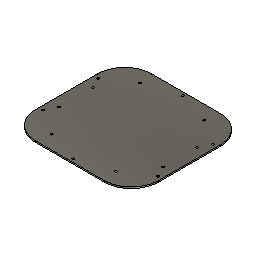
バスケット底 v3 (Autodesk Fusion 360 design; units mm, degrees)
Autodesk Fusion 360 part; units mm, degrees
note: some values were not read from the file. Set by a fixed rule: which sketch regions a step uses.
sketch "スケッチ1" plane through (0, 0, 0) normal (0, 0, 1) x (1, 0, 0)
  circle A0 centre (0, 0) radius 75
  circle A1 centre (0, 0) radius 85
  line L0 (0, 75) -> (0, 85)
  circle A2 centre (0, 80) radius 1.6
  circle A3 centre (-47.0228, 64.7214) radius 1.6
  circle A4 centre (-76.0845, 24.7214) radius 1.6
  circle A5 centre (-76.0845, -24.7214) radius 1.6
  circle A6 centre (-47.0228, -64.7214) radius 1.6
  circle A7 centre (0, -80) radius 1.6
  circle A8 centre (47.0228, -64.7214) radius 1.6
  circle A9 centre (76.0845, -24.7214) radius 1.6
  circle A10 centre (76.0845, 24.7214) radius 1.6
  circle A11 centre (47.0228, 64.7214) radius 1.6
  line L1 (0, 0) -> (-84, 0)
  line L2 (-84, 0) -> (-84, -40.186)
  line L3 (0, 0) -> (0, 85)
  line L4 (84, 0) -> (84, -40.186)
  line L5 (-84, 0) -> (-84, 40.186)
  line L6 (84, 0) -> (84, 40.186)
  circle A12 centre (-84, 40.186) radius 1.6
  circle A13 centre (84, 40.186) radius 1.6
  circle A14 centre (-84, -40.186) radius 1.6
  circle A15 centre (84, -40.186) radius 1.6
  line L7 (0, 85) -> (-90, 85)
  line L8 (-90, 85) -> (-90, 0)
  line L9 (-90, 0) -> (0, 0)
  line L10 (0, 0) -> (0, 85)
  line L11 (90, 85) -> (90, 0)
  line L12 (0, 85) -> (90, 85)
  line L13 (-90, -85) -> (-90, 0)
  line L14 (0, -85) -> (-90, -85)
  line L15 (0, -85) -> (90, -85)
  line L16 (90, -85) -> (90, 0)
  dimension "d1" = 150
  dimension "d4" = 170
  dimension "d7" = 3.2
  dimension "d9" = 360
  dimension "d10" = 84
  dimension "d11" = 40.186
  dimension "d12" = 3.2
  dimension "d13" = 3.2
  dimension "d14" = 3.2
  dimension "d15" = 3.2
  constraint coincident A0.centre A1.centre
  constraint concentric A0 A1
  constraint coincident A0 L0.start
  constraint coincident A1 L0.end
  constraint vertical L0
  constraint midpoint L0 A2.centre
  constraint horizontal L1
  constraint perpendicular L1 L2
  constraint parallel L0 L3
  constraint symmetric L1.end L3 L4.start
  constraint symmetric L2.end L3 L4.end
  constraint symmetric L2.start L1 L5.start
  constraint symmetric L1 L2.end L5.end
  constraint symmetric L1 L4.start L6.start
  constraint symmetric L1 L4.end L6.end
  constraint coincident L5.end A12.centre
  constraint coincident L6.end A13.centre
  constraint coincident L2.end A14.centre
  constraint coincident L4.end A15.centre
  constraint horizontal L7
  constraint vertical L8
  constraint horizontal L9
  constraint vertical L10
  constraint symmetric L0.end L3 L7.start
  constraint symmetric L3 L7.end L11.start
  constraint symmetric L3 L8.end L11.end
  constraint symmetric L0.end L9 L14.start
  constraint symmetric L7.end L9 L13.start
  constraint symmetric L8.end L9 L13.end
  constraint symmetric L9 L11.start L15.end
  constraint symmetric L9 L11.end L16.end
  constraint symmetric L9 L0.end L14.start
  measures "d1" diameter of A0
  measures "d4" diameter of A1
  measures "d7" diameter of A2
  measures "d10" distance of A0.centre L1.end
  measures "d11" distance of L1.end L2.end
  measures "d12" diameter of A12
  measures "d13" diameter of A13
  measures "d14" diameter of A14
  measures "d15" diameter of A15
extrude "押し出し1" add sketch "スケッチ1" along normal blind 2 contours A0 L1 L3 L9 L10 | A0 A1 L0 A2 L1 L2 L3 L4 L6 L9 L10 | A0 L1 L3 L9 L10 | A0 A1 L0 A2 L1 L3 L5 L9 L10 | A1 L5 L9 | A1 L2 L9 | A1 L9 L13 L14 | A1 L7 L8 L9 | A1 L11 L12 L15 L16 | A1 L4 L6
fillet "フィレット1" radius 40 4 edges at (-90, -85, 1) (90, -85, 1) (90, 85, 1) (-90, 85, 1)
equation "d10 = ( 168 / 2 ) * 1 mm"
equation "d11 = ( 80.372 / 2 ) * 1 mm"
